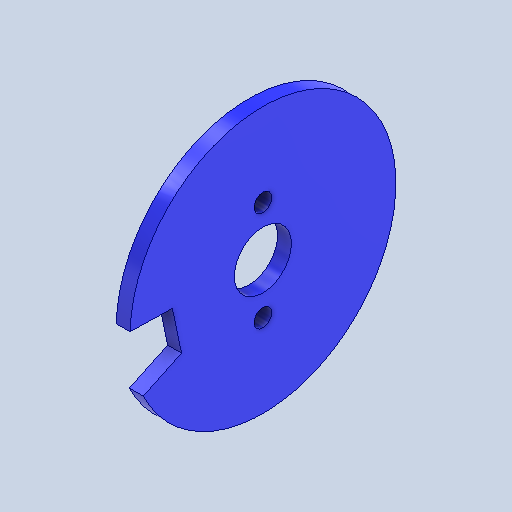
# Autodesk Inventor part: belt_liner_v2_3DP_P-4-F
Saved by Autodesk Inventor 2025.2 (Build 292293000, 293)
## iProperties
Created: 2025-01-13
Part Number: belt_liner_v2_3DP_P-4-F
Material: ABS プラスチック
Document SubType Name: Modeling
Designer: haruy
Density: 1.06 g/cm^3
Appearance: 青 - 壁塗料 - 光沢
Author: haruy
Autodesk Inventor part; units mm, degrees
ref_plane "YZ Plane" through (0, 0, 0) normal (1, 0, 0) x (0, 1, 0)
ref_plane "XZ Plane" through (0, 0, 0) normal (0, 1, 0) x (-1, 0, 0)
ref_plane "XY Plane" through (0, 0, 0) normal (0, 0, 1) x (1, 0, 0)
sketch "スケッチ2" plane through (0, 0, 0) normal (1, 0, 0) x (0, 1, 0)
  line L0 (-7.071, 15.2913) -> (-10.3324, 22.2065)
  arc A0 (-10.3324, 22.2065) -> (0.9209, 24.5984) centre (0.1387, 0.6112) ccw
  line L1 (0.9209, 24.5984) -> (0.7542, 16.9546)
  line L2 (0.7542, 16.9546) -> (-7.071, 15.2913)
  circle A1 centre (-8.8613, 0.6112) radius 1.6
  circle A2 centre (9.1387, 0.6112) radius 1.6
  circle A3 centre (0.1387, 0.6112) radius 5.15
  point P0 (0, 0)
  constraints: 6 end point, 4 centre point, 2 point on circle
extrude "押し出し2" add sketch "スケッチ2" along normal blind 2.5
